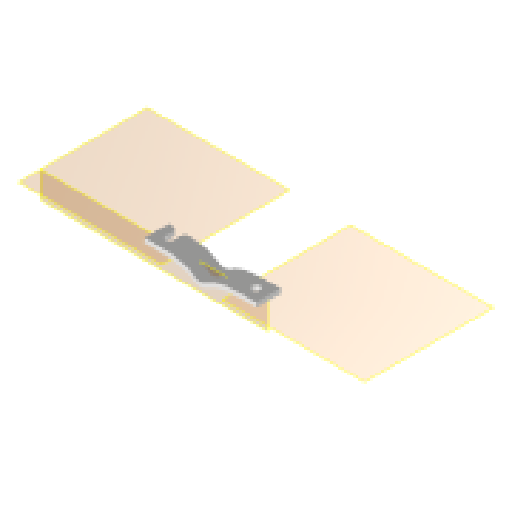
# Autodesk Inventor part: 60_Planktoscope_Sampleholder_2
Saved by Autodesk Inventor 2024.1 (Build 281209000, 209)
## iProperties
Created: 2024-06-28
Part Number: 60_Planktoscope_Sampleholder_2
Material: Generisch
Document SubType Name: Modeling
Designer: diederichbenedict
Density: 1 g/cm^3
Appearance: Vorgabe
Author: diederichbenedict
Autodesk Inventor part; units mm, degrees
ref_plane "YZ Plane" through (0, 0, 0) normal (1, 0, 0) x (0, 1, 0)
ref_plane "XZ Plane" through (0, 0, 0) normal (0, 1, 0) x (-1, 0, 0)
ref_plane "XY Plane" through (0, 0, 0) normal (0, 0, 1) x (1, 0, 0)
ref_plane "Arbeitsebene1" through (-42.5, -18.05, -10) normal (0, -1, 0) x (1, 0, 0)
sketch "Skizze1" plane through (-42.5, -18.05, -10) normal (0, -1, 0) x (1, 0, 0)
  line L0 (45.91, 10.609) -> (59.4818, 10.609) construction
  line L1 (59.4818, 10.609) -> (63.5906, 10.303) construction
  line L2 (63.5906, 10.303) -> (66.1223, 6.4827) construction
  line L3 (66.1223, 6.4827) -> (69.15, 6.4827) construction
  spline S0 degree 4 poles (45.91, 10.609) (59.4818, 10.609) (63.5906, 10.303) (66.1223, 6.4827) (69.15, 6.4827) knots 1 1 1 1 1 2 2 2 2 2
  line L4 (46.0094, 12.5239) -> (59.5812, 12.5239) construction
  line L5 (59.5812, 12.5239) -> (63.69, 12.218) construction
  line L6 (63.69, 12.218) -> (66.2218, 8.3976) construction
  line L7 (66.2218, 8.3976) -> (69.15, 8.1737) construction
  spline S1 degree 4 poles (46.0094, 12.5239) (59.5812, 12.5239) (63.69, 12.218) (66.2218, 8.3976) (69.15, 8.1737) knots 1 1 1 1 1 2 2 2 2 2
  line L8 (46.0094, 12.5239) -> (45.91, 10.609)
  line L9 (69.15, 8.1737) -> (69.15, 6.4827)
  line L10 (42.5, 16.2648) -> (42.5, 4.43) projected
  point P0 (54.5567, 11.9133)
  constraints: 4 end point, 1 parallel, 6 other
extrude "Extrusion1" add sketch "Skizze1" along normal mid plane 10
ref_plane "Arbeitsebene2" through (0, 0, 0) normal (0, 0, 1) x (1, 0, 0)
sketch "Skizze2" plane through (0, 0, 0) normal (0, 0, 1) x (1, 0, 0)
  line L0 (12.3, -18.05) -> (-2.05, -18.05) projected
  circle A0 centre (8.65, -14) radius 1.4 projected
  circle A1 centre (8.65, -18.05) radius 1.6
  point P0 (0, 0)
  dimension "d2" = 3.2
  constraints: 1 centre point, 1 point on line
  measures "d2" diameter of A1
extrude "Extrusion2" cut sketch "Skizze2" along normal mid plane 10 contours A1 L0 | L0 A1
mirror "Spiegeln1" about plane through (26.65, -18.05, -3.5173) normal (1, 0, 0) of "Extrusion1", "Extrusion2"
sketch "Skizze3" plane through (0, 0, 0) normal (0, 0, 1) x (1, 0, 0)
  line L0 (10.2456, -18.1688) -> (7.1543, -18.1688)
  line L1 (7.1543, -18.1688) -> (7.1543, 0.1733)
  line L2 (7.1543, 0.1733) -> (10.2456, 0.1733)
  line L3 (10.2456, 0.1733) -> (10.2456, -18.1688)
  point P0 (0, 0)
  constraints: 8 end point, 2 parallel, 1 horizontal, 1 perpendicular, 2 other
extrude "Extrusion3" cut sketch "Skizze3" along normal mid plane 10
fillet "Rundung1" radius 2 2 edges at (10.2456, -13.05, 1.4929) (7.1543, -13.05, 1.5517)
ref_plane "Arbeitsebene3" through (53.3, 0, 0) normal (0, 0, -1) x (-1, 0, 0)
